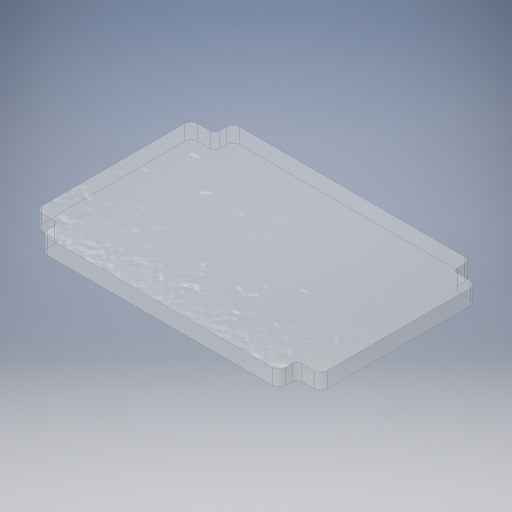
# Autodesk Inventor part: BT702_trajan20_21
Saved by Autodesk Inventor 2023 (Build 270158000, 158)
## iProperties
Company: HTBLA Kaindorf
RuleStatus: InUse
Created: 2022-08-21
Part Number: BT702_trajan20_21
Project: Zeichenmaschine_v2
Material: Acryl
Description: Plexi_40x80
Document SubType Name: Modeling
Designer: trajan20
Density: 1.188 g/cm^3
Appearance: Transparent - farblos
Mass: 32.5152 g
Surface Area: 124.347 cm^2
Volume: 27.3697 cm^3
AfterDocNew0: iProperties-Editor_aufrufen
Author: jan
Keywords: 2021
Autodesk Inventor part; units mm, degrees
ref_plane "YZ Plane" through (0, 0, 0) normal (1, 0, 0) x (0, 1, 0)
ref_plane "XZ Plane" through (0, 0, 0) normal (0, 1, 0) x (-1, 0, 0)
ref_plane "XY Plane" through (0, 0, 0) normal (0, 0, 1) x (1, 0, 0)
sketch "Skizze3" plane through (0, 0, 0) normal (0, 0, 1) x (1, 0, 0)
  line L0 (0, 0) -> (-50, 0)
  line L1 (-50, 0) -> (-50, 80)
  line L2 (-50, 80) -> (0, 80)
  line L3 (0, 80) -> (0, 0)
  line L4 (-50, 78.2) -> (-55.85, 78.2)
  line L5 (-55.85, 78.2) -> (-55.85, 40)
  line L6 (-55.85, 40) -> (-50, 40)
  line L7 (-50, 40) -> (-50, 78.2)
  line L8 (-50, 80) -> (-25, 80)
  line L9 (-25, 80) -> (-25, 85.85)
  line L10 (-25, 85.85) -> (-50, 85.85)
  line L11 (-50, 85.85) -> (-50, 80)
  dimension "d4" = 80
  dimension "d5" = 50
  dimension "d6" = 5.85
  dimension "d7" = 1.8
  dimension "d8" = 5.85
  constraints: 24 end point, 6 parallel, 3 horizontal, 3 perpendicular, 3 point on line, 2 midpoint
  measures "d4" distance between parallel lines of L2 L0
  measures "d5" distance between parallel lines of L1 L3
  measures "d6" distance between parallel lines of L2 L10
  measures "d7" distance between parallel lines of L2 L4
  measures "d8" distance between parallel lines of L1 L5
extrude "Extrusion3" add sketch "Skizze3" along normal blind 5 contours L0 L1 L2 L3
extrude "Extrusion4" add sketch "Skizze3" along normal blind 5 contours L6 L5 L4 L1 | L2 L11 L10 L9
fillet "Rundung1" radius 2 2 edges at (-55.85, 78.2, 2.5) (-50, 85.85, 2.5)
mirror "Spiegeln1" about plane through (-55.85, 40, 0) normal (0, -1, 0) of "Extrusion4", "Rundung1"
mirror "Spiegeln2" about plane through (-25, 80, 0) normal (1, 0, 0) of "Extrusion4", "Rundung1", "Spiegeln1"
fillet "Rundung2" radius 1.5 4 edges at (0, 78.2, 2.5) (-50, 78.2, 2.5) (-50, 1.8, 2.5) (0, 1.8, 2.5)
derived "BT000_trajan20_22_Zeichenmaschine_neu_Masterskizze.ipt"
equation "\"d4\" = Basis_Haupt_Höhe_Profillänge - 4 * AluProfil_Abstand"
equation "\"d5\" = -2 * AluProfil_Abstand + 0.5 * Basis_Haupt_Länge_Profillänge - 0.5 * Basis_Zubau_Breite_Profillänge"
equation "\"d6\" = d8"
equation "\"Basis_Haupt_Höhe_Profillänge\" = 120"
equation "\"AluProfil_Abstand\" = 10"
equation "\"Basis_Haupt_Länge_Profillänge\" = 220"
equation "\"Basis_Zubau_Breite_Profillänge\" = 80"
